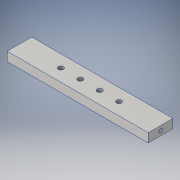
# Autodesk Inventor part: Kühkörper_GateTreiber
Saved by Autodesk Inventor 2016 (Build 200138000, 138)
## iProperties
Created: 2018-05-17
Part Number: Kühkörper_GateTreiber
Material: Aluminum 6061
Document SubType Name: Modeling
Designer: Phil Erle
Density: 2.7 g/cm^3
Appearance: Aluminum - Flat
Author: Phil Erle
Autodesk Inventor part; units mm, degrees
ref_plane "YZ Plane" through (0, 0, 0) normal (1, 0, 0) x (0, 1, 0)
ref_plane "XZ Plane" through (0, 0, 0) normal (0, 1, 0) x (-1, 0, 0)
ref_plane "XY Plane" through (0, 0, 0) normal (0, 0, 1) x (1, 0, 0)
sketch "Sketch1" plane through (0, 0, 0) normal (0, 0, 1) x (1, 0, 0)
  line L0 (-47.25, -8.25) -> (47.25, -8.25)
  line L1 (47.25, -8.25) -> (47.25, 8.25)
  line L2 (47.25, 8.25) -> (-47.25, 8.25)
  line L3 (-47.25, 8.25) -> (-47.25, -8.25)
  line L4 (-47.25, -8.25) -> (47.25, 8.25) construction
  line L5 (47.25, -8.25) -> (-47.25, 8.25) construction
  point P0 (0, 0)
  dimension "d0" = 94.5
  dimension "d1" = 16.5
  constraints: 12 end point, 2 midpoint, 2 parallel, 1 horizontal, 1 perpendicular
  measures "d0" distance of L2.end L1.end
  measures "d1" distance of L0.end L1.end
extrude "Extrusion1" add sketch "Sketch1" along normal blind 6
sketch "Sketch2" plane through (0, 0, 6) normal (0, 0, 1) x (1, 0, 0)
  line L0 (-19.5, 0) -> (-6.5, 0) construction
  line L1 (6.5, 0) -> (-6.5, 0) construction
  line L2 (6.5, 0) -> (19.5, 0) construction
  point P0 (0, 0)
  point P1 (0, 0)
  dimension "d4" = 13
  dimension "d5" = 13
  dimension "d6" = 13
  constraints: 6 end point, 2 horizontal, 1 coincident, 1 collinear, 1 horizontal alignment, 1 midpoint
  measures "d4" distance of L0.start L0.end
  measures "d5" distance of L1.start L0.end
  measures "d6" distance of L1.start L2.end
hole "Hole1" at (-19.5, 0, 6) at (-6.5, 0, 6) at (6.5, 0, 6) at (19.5, 0, 6) direction (0, 0, -1) diameter 3.4 depth 8 tip angle 118 clearance for "Countersunk Flat Head Screw DIN EN ISO 2009" size "M3" standard "DIN"
sketch "Sketch3" plane through (47.25, -8.25, 0) normal (1, 0, 0) x (0, 0, -1)
  line L0 (0, 0) -> (0, 16.5) projected
  point P0 (0, 8.25)
  point P1 (-3, 8.25)
  point P2 (0, 8.25)
  dimension "d14" = 3
  constraints: 1 horizontal alignment, 1 midpoint
  measures "d14" horizontal distance of L0.start point (-3, 8.25)
hole "Hole2" at (47.25, 0, 3) direction (-1, 0, 0) diameter 2.459 depth 8.8 tip angle 118 thread size "M3x0.5" class "6H" standard "ISO Metric profile"
body "Solid1"
